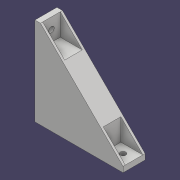
# Autodesk Inventor part: L Bracket Small
Saved by Autodesk Inventor 2017 SP1 (Build 210196100, 196)
## iProperties
Created: 2018-05-02
Part Number: L Bracket Small
Material: Generic
Document SubType Name: Modeling
Designer: Zach
Density: 1 g/cm^3
Appearance: Default
Author: Zach
Autodesk Inventor part; units mm, degrees
ref_plane "YZ Plane" through (0, 0, 0) normal (1, 0, 0) x (0, 1, 0)
ref_plane "XZ Plane" through (0, 0, 0) normal (0, 1, 0) x (-1, 0, 0)
ref_plane "XY Plane" through (0, 0, 0) normal (0, 0, 1) x (1, 0, 0)
sketch "Sketch1" plane through (0, 0, 0) normal (0, 0, 1) x (1, 0, 0)
  line L0 (0, 0) -> (80, 0)
  line L1 (80, 0) -> (80, 20)
  line L2 (80, 20) -> (0, 20)
  line L3 (0, 20) -> (0, 0)
  circle A0 centre (70, 10) radius 2.5
  point P0 (80, 10)
  dimension "d0" = 80
  dimension "d1" = 20
  dimension "d2" = 5
  dimension "d3" = 10
  constraints: 8 end point, 2 parallel, 1 centre point, 1 horizontal, 1 horizontal alignment, 1 midpoint, 1 perpendicular
  measures "d0" distance of L2.end L1.end
  measures "d1" distance of L1.end L0.end
  measures "d2" diameter of A0
  measures "d3" distance from line of L1 A0.centre
extrude "Extrusion1" add sketch "Sketch1" along normal blind 5
sketch "Sketch2" plane through (0, 0, 0) normal (-1, 0, 0) x (0, 0, 1)
  line L0 (0, 0) -> (0, 20) projected
  line L1 (0, 20) -> (80, 20)
  line L2 (80, 20) -> (80, 0)
  line L3 (80, 0) -> (0, 0)
  line L4 (0, 0) -> (0, 20)
  circle A0 centre (70, 10) radius 2.5
  point P0 (5, 0)
  point P1 (80, 10)
  dimension "d6" = 80
  dimension "d7" = 5
  dimension "d8" = 10
  constraints: 8 end point, 2 parallel, 1 centre point, 1 horizontal, 1 horizontal alignment, 1 midpoint, 1 perpendicular, 1 point on line
  measures "d6" distance of L2.end L3.end
  measures "d7" diameter of A0
  measures "d8" distance from line of L2 A0.centre
extrude "Extrusion2" add sketch "Sketch2" against normal blind 5
sketch "Sketch3" plane through (0, 20, 0) normal (0, 1, 0) x (1, 0, 0)
  line L0 (80, -5) -> (5, -5) projected
  line L1 (5, -5) -> (5, -80) projected
  line L2 (5, -80) -> (5, -5) projected
  line L3 (5, -80) -> (80, -5)
  point P0 (0, 0)
  constraints: 2 end point
extrude "Extrusion3" add sketch "Sketch3" against normal blind 2
sketch "Sketch4" plane through (0, 0, 0) normal (0, -1, 0) x (1, 0, 0)
  line L0 (80, 5) -> (5, 5) projected
  line L1 (80, 5) -> (5, 80) projected
  line L2 (5, 5) -> (5, 80) projected
  point P0 (0, 0)
extrude "Extrusion4" add sketch "Sketch4" against normal blind 2
sketch "Sketch5" plane through (0, 18, 0) normal (0, -1, 0) x (1, 0, 0)
  line L0 (5, 72.5) -> (5, 67.5) projected
  line L1 (67.5, 5) -> (72.5, 5) projected
  line L2 (5, 67.5) -> (5, 5)
  line L3 (5, 5) -> (67.5, 5)
  line L4 (5, 60) -> (60, 5)
  line L5 (70, 5) -> (70, 0)
  line L6 (80, 0) -> (0, 0) projected
  line L7 (5, 70) -> (0, 70)
  line L8 (5, 60) -> (25, 60)
  line L9 (60, 5) -> (60, 25)
  line L10 (5, 80) -> (80, 5) projected
  line L11 (25, 60) -> (60, 25)
  dimension "d15" = 10
  dimension "d16" = 10
  constraints: 16 end point, 5 point on line, 3 vertical, 2 horizontal, 2 midpoint, 1 collinear, 1 perpendicular
  measures "d15" distance from line of L4.start L7
  measures "d16" distance of L4.end L5.start
extrude "Extrusion5" add sketch "Sketch5" along normal blind 16
body "Solid1"
